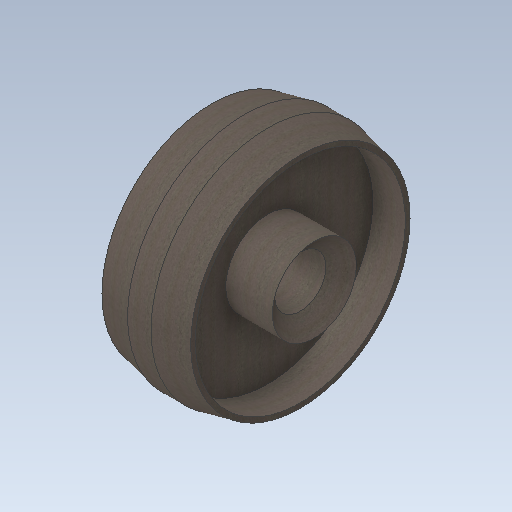
# Autodesk Inventor part: wheel
Saved by Autodesk Inventor 2020 (Build 240168000, 168)
## iProperties
Created: 2021-06-13
Part Number: wheel
Material: Steel, Carbon
Document SubType Name: Modeling
Designer: joelm
Density: 7.85 g/cm^3
Appearance: Walnut
Mass: 985.819 g
Surface Area: 404.587 cm^2
Volume: 125.582 cm^3
Author: joelm
Autodesk Inventor part; units mm, degrees
ref_plane "YZ Plane" through (0, 0, 0) normal (1, 0, 0) x (0, 1, 0)
ref_plane "XZ Plane" through (0, 0, 0) normal (0, 1, 0) x (-1, 0, 0)
ref_plane "XY Plane" through (0, 0, 0) normal (0, 0, 1) x (1, 0, 0)
sketch "Sketch1" plane through (0, 0, 0) normal (0, 0, 1) x (1, 0, 0)
  line L0 (0, 0) -> (50, 0)
  line L1 (6, 11) -> (44, 11)
  line L2 (20, 50) -> (30, 50)
  line L3 (20, 18) -> (20, 45)
  line L4 (30, 18) -> (30, 45)
  line L5 (0, 18) -> (20, 18)
  line L6 (30, 18) -> (50, 18)
  line L7 (44, 45) -> (44, 47)
  line L8 (6, 45) -> (6, 47)
  line L9 (44, 47) -> (30, 50)
  line L10 (20, 50) -> (6, 47)
  line L11 (6, 45) -> (20, 45)
  line L12 (30, 45) -> (44, 45)
  line L13 (50, 18) -> (44, 11)
  line L14 (6, 11) -> (0, 18)
  dimension "d0" = 50
  dimension "d2" = 38
  dimension "d3" = 11
  dimension "d4" = 39
  dimension "d8" = 10
  dimension "d9" = 20
  dimension "d12" = 2
  dimension "d13" = 2
  dimension "d14" = 18
  dimension "d15" = 26.2486
  dimension "d16" = 11.7142
  dimension "d17" = 18
  dimension "d18" = 45
  constraints: 30 end point, 6 parallel, 2 horizontal, 2 vertical
  measures "d0" distance of L0.start L0.end
  measures "d2" distance of L1.start L1.end
  measures "d3" vertical distance of L1.start L0.start
  measures "d4" distance between parallel lines of L1 L2
  measures "d8" distance between parallel lines of L3 L4
  measures "d9" distance from line of L3 L0.start
  measures "d12" distance of L7.start L7.end
  measures "d13" distance of L8.start L8.end
  measures "d14" distance from line of L0.start L6
  measures "d15" distance from line of L0.start L13
  measures "d16" distance from line of L0.start L14
  measures "d17" distance from line of L0.start L5
  measures "d18" distance from line of L0.start L12
revolve "Revolution1" add sketch "Sketch1" angle 360 about axis through (0, 0, 0) along (1, 0, 0)
body "Solid1"
